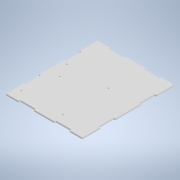
# Autodesk Inventor part: Base
Saved by Autodesk Inventor 2020.3 (Build 243373000, 373)
## iProperties
Created: 2020-08-22
Part Number: Base
Material: Generic
Document SubType Name: Modeling
Designer: Scott Hanson
Density: 1 g/cm^3
Appearance: Default
Author: Scott Hanson
Autodesk Inventor part; units mm, degrees
ref_plane "YZ Plane" through (0, 0, 0) normal (1, 0, 0) x (0, 1, 0)
ref_plane "XZ Plane" through (0, 0, 0) normal (0, 1, 0) x (-1, 0, 0)
ref_plane "XY Plane" through (0, 0, 0) normal (0, 0, 1) x (1, 0, 0)
sketch "Sketch1" plane through (0, 0, 0) normal (0, 1, 0) x (-1, 0, 0)
  line L0 (0, 0) -> (-150, 0)
  line L1 (-150, 0) -> (-150, -180)
  line L2 (-150, -180) -> (0, -180)
  line L3 (0, -180) -> (0, 0)
  dimension "d0" = 180
  dimension "d1" = 150
  constraints: 8 end point, 2 parallel, 1 horizontal, 1 perpendicular
  measures "d0" distance of L2.end L0.start
  measures "d1" distance of L0.start L0.end
extrude "Baseplate" add sketch "Sketch1" along normal blind 3
sketch "TabsSketch" plane through (0, 3, 0) normal (0, 1, 0) x (1, 0, 0)
  line L0 (0, 180) -> (0, 0) projected
  line L1 (0, 35) -> (3, 35)
  line L2 (3, 35) -> (3, 65)
  line L3 (3, 65) -> (0, 65)
  line L4 (0, 65) -> (0, 35)
  line L5 (0, 115) -> (3, 115)
  line L6 (3, 115) -> (3, 145)
  line L7 (3, 145) -> (0, 145)
  line L8 (0, 145) -> (0, 115)
  line L9 (0, 0) -> (150, 0) projected
  line L10 (150, 180) -> (0, 180) projected
  line L11 (75, 0) -> (75, 180) construction
  line L12 (25, 0) -> (55, 0)
  line L13 (55, 0) -> (55, 3)
  line L14 (55, 3) -> (25, 3)
  line L15 (25, 3) -> (25, 0)
  line L16 (25, 180) -> (55, 180)
  line L17 (55, 180) -> (55, 177)
  line L18 (55, 177) -> (25, 177)
  line L19 (25, 177) -> (25, 180)
  line L20 (150, 180) -> (150, 0)
  line L21 (150, 35) -> (147, 35)
  line L22 (147, 35) -> (147, 65)
  line L23 (147, 65) -> (150, 65)
  line L24 (150, 65) -> (150, 35)
  line L25 (150, 115) -> (147, 115)
  line L26 (147, 115) -> (147, 145)
  line L27 (147, 145) -> (150, 145)
  line L28 (150, 145) -> (150, 115)
  line L29 (150, 0) -> (0, 0)
  line L30 (0, 180) -> (150, 180)
  line L31 (125, 0) -> (95, 0)
  line L32 (95, 0) -> (95, 3)
  line L33 (95, 3) -> (125, 3)
  line L34 (125, 3) -> (125, 0)
  line L35 (125, 180) -> (95, 180)
  line L36 (95, 180) -> (95, 177)
  line L37 (95, 177) -> (125, 177)
  line L38 (125, 177) -> (125, 180)
  point P0 (0, 65)
  dimension "d4" = 3
  dimension "d5" = 35
  dimension "d7" = 35
  dimension "d8" = 30
  dimension "d9" = 30
  dimension "d10" = 50
  dimension "d11" = 3
  dimension "d12" = 3
  dimension "d13" = 30
  dimension "d14" = 30
  dimension "d15" = 25
  dimension "d16" = 40
  constraints: 72 end point, 20 symmetric about line, 12 point on line, 8 parallel, 4 horizontal, 4 perpendicular, 2 midpoint
  measures "d4" distance of L1.start L1.end
  measures "d5" distance from line of L1.end L9
  measures "d7" distance from line of L10 L6.end
  measures "d8" distance of L5.end L6.end
  measures "d9" distance of L1.end L2.end
  measures "d10" distance of L5.end L2.end
  measures "d11" distance of L12.start L14.end
  measures "d12" distance of L18.end L16.start
  measures "d13" distance of L13.end L14.end
  measures "d14" distance of L17.end L18.end
  measures "d15" distance from line of L18.end L0
  measures "d16" distance of L37.start L17.end
extrude "Extrusion2" cut sketch "TabsSketch" against normal through all contours L7 L6 L5 L0 | L10 L17 L18 L19 | L3 L2 L1 L0 | L10 L38 L37 L36 | L15 L14 L13 L9 | L20 L25 L26 L27 | L32 L33 L34 L9 | L20 L21 L22 L23
sketch "Sketch3" plane through (0, 3, 0) normal (0, 1, 0) x (1, 0, 0)
  circle A0 centre (10, 20) radius 1.6
  circle A1 centre (10, 109.5) radius 1.6
  circle A2 centre (91.5, 20) radius 1.6
  circle A3 centre (91.5, 109.5) radius 1.6
  line L0 (0, 35) -> (0, 0) projected
  line L1 (0, 115) -> (0, 65) projected
  line L2 (0, 0) -> (25, 0) projected
  line L3 (55, 0) -> (95, 0) projected
  circle A4 centre (23.5, 81.5) radius 1.6
  dimension "d19" = 3.2
  dimension "d20" = 3.2
  dimension "d21" = 3.2
  dimension "d22" = 3.2
  dimension "d23" = 89.5
  dimension "d24" = 81.5
  dimension "d25" = 89.5
  dimension "d26" = 81.5
  dimension "d27" = 10
  dimension "d28" = 10
  dimension "d29" = 20
  dimension "d30" = 20
  dimension "d31" = 61.5
  dimension "d32" = 68
  dimension "d33" = 3.2
  constraints: 5 centre point
  measures "d19" diameter of A0
  measures "d20" diameter of A1
  measures "d21" diameter of A2
  measures "d22" diameter of A3
  measures "d23" distance of A1.centre A0.centre
  measures "d24" distance of A2.centre A0.centre
  measures "d25" distance of A3.centre A2.centre
  measures "d26" distance of A1.centre A3.centre
  measures "d27" distance from line of A0.centre L0
  measures "d28" distance from line of A1.centre L1
  measures "d29" distance from line of A0.centre L2
  measures "d30" distance from line of A2.centre L3
  measures "d31" vertical distance of A4.centre A2.centre
  measures "d32" horizontal distance of A4.centre A2.centre
  measures "d33" diameter of A4
extrude "PCB Mounting" cut sketch "Sketch3" against normal through all
equation "\"d7\" = d5"
equation "\"d8\" = d9"
equation "\"d12\" = d11"
equation "\"d13\" = d9"
equation "\"d14\" = d13"
equation "\"d20\" = d19"
equation "\"d21\" = d19"
equation "\"d22\" = d20"
equation "\"d25\" = d23"
equation "\"d26\" = d24"
equation "\"d28\" = d27"
equation "\"d30\" = d29"
body "Solid1"
